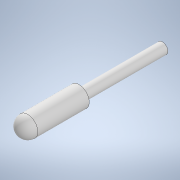
# Autodesk Inventor part: SpringRod
Saved by Autodesk Inventor 2022 (Build 260153000, 153)
## iProperties
Created: 2021-10-24
Part Number: SpringRod
Material: Generic
Document SubType Name: Modeling
Designer: teh18
Density: 1 g/cm^3
Appearance: Default
Author: teh18
Autodesk Inventor part; units mm, degrees
ref_plane "YZ Plane" through (0, 0, 0) normal (1, 0, 0) x (0, 1, 0)
ref_plane "XZ Plane" through (0, 0, 0) normal (0, 1, 0) x (-1, 0, 0)
ref_plane "XY Plane" through (0, 0, 0) normal (0, 0, 1) x (1, 0, 0)
sketch "Sketch1" plane through (0, 0, 0) normal (0, 0, 1) x (1, 0, 0)
  circle A0 centre (0, 0) radius 6
  dimension "d0" = 12
  constraints: 1 centre point, 1 coincident
  measures "d0" diameter of A0
extrude "Extrusion1" add sketch "Sketch1" along normal blind 24.38 and the other way blind 10
fillet "Fillet1" radius 6 1 edges at (-6, 0, 24.38)
sketch "Sketch2" plane through (0, 0, -10) normal (0, 0, -1) x (-1, 0, 0)
  circle A0 centre (0, 0) radius 3.4
  dimension "d6" = 6.8
  constraints: 1 centre point, 1 coincident
  measures "d6" diameter of A0
extrude "Extrusion2" add sketch "Sketch2" along normal blind 46
thicken "Thicken1" operation add thickness 0.4 both sides no extend neighbours yes toward (-0.9870503, 0.1604113, 0) faces at (5.9223, -0.9625, 12.2533) (5.9223, -0.9625, -6.6667) (-5.8689, 0, 19.6275)
thicken "Thicken2" operation add thickness 0.4 both sides no extend neighbours yes toward (0.9967573, -0.0804666, 0) faces at (-3.389, 0.2736, -25.3333)
body "Solid1"
